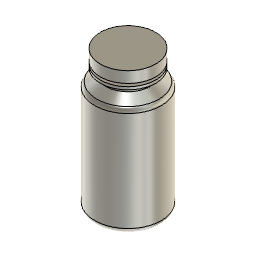
nalgene (Autodesk Fusion 360 design; units mm, degrees)
Autodesk Fusion 360 part; units mm, degrees
sketch "Sketch1" plane through (0, 0, 0) normal (0, 1, 0) x (1, 0, 0)
  line L0 (0, 0) -> (0, -25)
  line L1 (0, 0) -> (5, 0)
  arc A0 (6, -1) -> (5, 0) centre (5, -1) ccw
  line L2 (6, -1) -> (6, -19)
  arc A1 (5.6, -19.8) -> (6, -19) centre (5, -19) ccw
  line L3 (0, -25) -> (5, -25)
  line L4 (5, -25) -> (5, -23)
  line L5 (5, -23) -> (4, -23)
  line L6 (4, -21) -> (5.6, -19.8)
  line L7 (4, -23) -> (4, -22.5)
  line L8 (4, -21) -> (4, -22)
  line L9 (4, -22.5) -> (5, -22.5)
  line L10 (5, -22.5) -> (5, -22)
  line L11 (5, -22) -> (4, -22)
  dimension "d1" = 25
  dimension "d2" = 5
  dimension "d3" = 18
  dimension "d4" = 5
  dimension "d5" = 2
  dimension "d6" = 1
  dimension "d7" = 2
  dimension "d8" = 0.5
  dimension "d9" = 1
  dimension "d10" = 1
  dimension "d11" = 0.5
  constraint coincident L0.start L1.start
  constraint vertical L0
  constraint perpendicular L0 L1
  constraint vertical L2
  constraint perpendicular L0 L3
  constraint perpendicular L3 L4
  constraint perpendicular L4 L5
  constraint tangent A1 L6
  constraint perpendicular L5 L7
  constraint vertical L8
  constraint perpendicular L7 L9
  constraint perpendicular L9 L10
  constraint perpendicular L8 L11
  measures "d1" distance of L0.start L0.end
  measures "d2" distance of L0.start L1.end
  measures "d3" distance of A0.start L2.end
  measures "d4" distance of L0.end L3.end
  measures "d5" distance of L3.end L4.end
  measures "d6" distance of L4.end L5.end
  measures "d7" distance of L5.end L6.start
  measures "d8" distance of L5.end L7.end
  measures "d9" distance of L6.start L8.end
  measures "d10" distance of L7.end L9.end
  measures "d11" distance of L9.end L10.end
revolve "Revolve1" add sketch "Sketch1" angle 360 about axis through (0, 0, 0) along (0, 0, 1)
